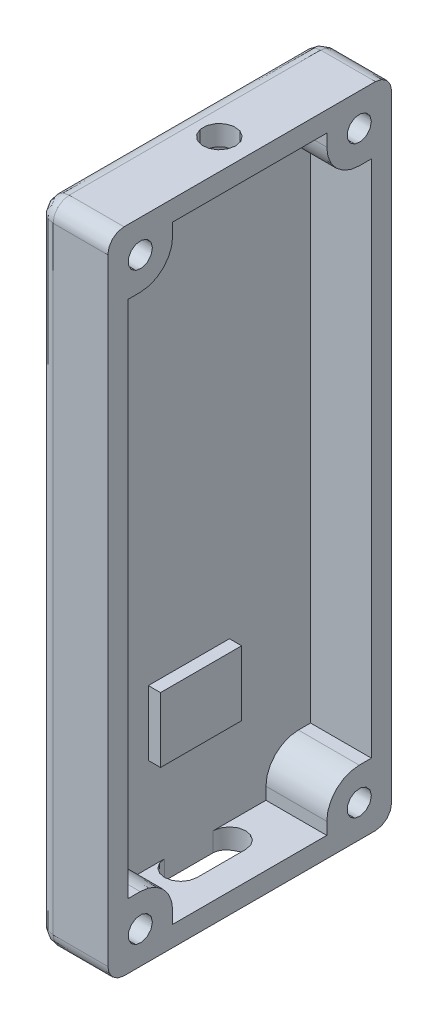
# Autodesk Inventor part: 111
Saved by Autodesk Inventor 2024 (Build 280153000, 153)
## iProperties
Created: 2025-04-29
Part Number: 111
Material: 일반
Document SubType Name: Modeling
Designer: User
Density: 1 g/cm^3
Appearance: 기본값
Author: User
Autodesk Inventor part; units mm, degrees
ref_plane "YZ Plane" through (0, 0, 0) normal (1, 0, 0) x (0, 1, 0)
ref_plane "XZ Plane" through (0, 0, 0) normal (0, 1, 0) x (-1, 0, 0)
ref_plane "XY Plane" through (0, 0, 0) normal (0, 0, 1) x (1, 0, 0)
sketch "스케치1" plane through (0, 0, 0) normal (1, 0, 0) x (0, 1, 0)
  line L0 (0, 0) -> (80, 0)
  line L1 (80, 0) -> (80, -35)
  line L2 (80, -35) -> (0, -35)
  line L3 (0, -35) -> (0, 0)
  dimension "d0" = 35
  dimension "d1" = 80
  constraints: 8 end point, 2 parallel, 1 horizontal, 1 perpendicular
  measures "d0" distance between parallel lines of L0 L2
  measures "d1" distance between parallel lines of L3 L1
extrude "돌출1" add sketch "스케치1" along normal blind 8.75
sketch "스케치2" plane through (8.75, 0, 0) normal (1, 0, 0) x (0, 0, -1)
  line L0 (35, 80) -> (0, 80) projected
  line L1 (35, 0) -> (35, 80) projected
  line L2 (0, 80) -> (0, 0) projected
  line L3 (0, 0) -> (35, 0) projected
  line L4 (2.5, 77.5) -> (32.5, 77.5)
  line L5 (32.5, 77.5) -> (32.5, 2.5)
  line L6 (32.5, 2.5) -> (2.5, 2.5)
  line L7 (2.5, 2.5) -> (2.5, 77.5)
  dimension "d4" = 2.5
  constraints: 8 end point, 3 other
  measures "d4" distance between parallel lines of L0 L4
extrude "돌출2" cut sketch "스케치2" against normal blind 7.5 contours L4 L5 L6 L7
sketch "스케치3" plane through (0, 0, -35) normal (0, -1, 0) x (1, 0, 0)
  line L0 (1.25, 22.5) -> (5.25, 22.5)
  line L1 (5.25, 22.5) -> (5.25, 12.5)
  line L2 (5.25, 12.5) -> (1.25, 12.5)
  line L3 (1.25, 12.5) -> (1.25, 22.5)
  line L4 (1.25, 2.5) -> (1.25, 32.5) projected
  line L5 (0, 0) -> (8.75, 0) projected
  line L6 (0, 35) -> (8.75, 35) projected
  circle A0 centre (3.25, 14.5) radius 2
  circle A1 centre (3.25, 20.5) radius 2
  point P0 (1.25, 14.5)
  point P1 (5.25, 14.5)
  point P2 (5.25, 20.5)
  point P3 (1.25, 20.5)
  dimension "d7" = 4
  dimension "d8" = 10
  dimension "d9" = 12.5
  dimension "d10" = 35
  constraints: 8 end point, 6 tangent, 2 centre point, 2 parallel, 1 collinear, 1 horizontal, 1 perpendicular
  measures "d7" distance between parallel lines of L1 L3
  measures "d8" distance between parallel lines of L0 L2
  measures "d9" distance between parallel lines of L2 L5
  measures "d10" distance between parallel lines of L5 L6
extrude "돌출3" cut sketch "스케치3" against normal blind 2.5 contours A1 | A1 L1 A0 L3 | A0
sketch "스케치6" plane through (1.25, 0, 0) normal (1, 0, 0) x (0, 0, -1)
  line L0 (12.5, 14) -> (22.5, 14)
  line L1 (22.5, 14) -> (22.5, 22)
  line L2 (22.5, 22) -> (12.5, 22)
  line L3 (12.5, 22) -> (12.5, 14)
  line L4 (14.5, 0) -> (12.5, 0) projected
  line L5 (22.5, 0) -> (20.5, 0) projected
  line L6 (20.5, 0) -> (14.5, 0) projected
  point P0 (0, 0)
  dimension "d22" = 14
  dimension "d23" = 8
  constraints: 8 end point, 2 parallel, 2 point on line, 1 horizontal, 1 perpendicular
  measures "d22" distance between parallel lines of L0 L6
  measures "d23" distance between parallel lines of L0 L2
extrude "돌출6" add sketch "스케치6" along normal blind 1.5
sketch "스케치4" plane through (8.75, 0, 0) normal (1, 0, 0) x (0, 0, -1)
  line L0 (35, 0) -> (27, 0)
  line L1 (27, 0) -> (27, 8)
  line L2 (27, 8) -> (35, 8)
  line L3 (35, 8) -> (35, 0)
  line L4 (0, 0) -> (8, 0)
  line L5 (8, 0) -> (8, 8)
  line L6 (8, 8) -> (0, 8)
  line L7 (0, 8) -> (0, 0)
  line L8 (0, 80) -> (8, 80)
  line L9 (8, 80) -> (8, 72)
  line L10 (8, 72) -> (0, 72)
  line L11 (0, 72) -> (0, 80)
  line L12 (35, 0) -> (35, 80) projected
  line L13 (35, 80) -> (27, 80)
  line L14 (27, 80) -> (27, 72)
  line L15 (27, 72) -> (35, 72)
  line L16 (35, 72) -> (35, 80)
  circle A0 centre (4, 76) radius 4
  circle A1 centre (31, 76) radius 4
  circle A2 centre (31, 4) radius 4
  circle A3 centre (4, 4) radius 4
  circle A4 centre (4, 4) radius 1.5
  circle A5 centre (31, 4) radius 1.5
  circle A6 centre (31, 76) radius 1.5
  circle A7 centre (4, 76) radius 1.5
  point P0 (8, 4)
  point P1 (4, 8)
  point P2 (31, 8)
  point P3 (27, 4)
  point P4 (4, 72)
  point P5 (8, 76)
  point P6 (27, 76)
  point P7 (31, 72)
  dimension "d14" = 8
  dimension "d16" = 3
  constraints: 32 end point, 12 tangent, 8 centre point, 8 parallel, 8 perpendicular, 4 coincident, 4 horizontal, 3 equal radius, 2 point on line, 1 collinear
  measures "d14" distance between parallel lines of L0 L2
  measures "d16" diameter of A5
extrude "돌출4" add sketch "스케치4" against normal up to next contours L0 A2 L3 | L0 L1 A2 | A2 | A2 L2 L3 | L7 A3 L4 | A3 L5 L4 | A3 | L7 L6 A3 | L8 A0 L11 | L8 L9 A0 | A0 | A0 L10 L11 | L15 A1 L12 | A1 L13 L12 | A1 | A1 L14 L13
sketch "스케치7" plane through (0, 80, 0) normal (0, 1, 0) x (1, 0, 0)
  circle A0 centre (5, 17.5) radius 2
  line L0 (0, 35) -> (8.75, 35) projected
  line L1 (0, 0) -> (8.75, 0) projected
  line L2 (0, 35) -> (0, 0) projected
  point P0 (-3.75, 35)
  point P1 (0, 27)
  dimension "d26" = 4
  dimension "d27" = 35
  dimension "d28" = 17.5
  dimension "d29" = 5
  constraints: 1 centre point
  measures "d26" diameter of A0
  measures "d27" distance between parallel lines of L0 L1
  measures "d28" distance from line of A0.centre L1
  measures "d29" distance from line of A0.centre L2
extrude "돌출7" cut sketch "스케치7" against normal blind 2.5
fillet "모깎기2" radius 2 8 edges at (4.375, 80, 0) (0, 80, -17.5) (0, 40, -35) (4.375, 0, -35) (0, 0, -17.5) (0, 40, 0) (4.375, 0, 0) (4.375, 80, -35)
equation "\"d9\" = -0.5 * d8 + 0.5 * d10"
equation "\"d28\" = 0.5 * d27"
